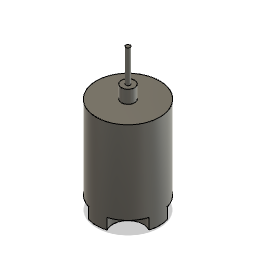
Motor v1 (Autodesk Fusion 360 design; units mm, degrees)
Autodesk Fusion 360 part; units mm, degrees
note: some values were not read from the file. Set by a fixed rule: which sketch regions a step uses.
sketch "Sketch1" plane through (0, 0, 0) normal (0, 1, 0) x (1, 0, 0)
  circle A0 centre (0, 0) radius 14.5
  dimension "d1" = 29
  constraint coincident A0.centre origin
  measures "d1" diameter of A0
extrude "Extrude1" add sketch "Sketch1" along normal blind 5
sketch "Sketch2" plane through (0, 0, 0) normal (0, -1, 0) x (1, 0, 0)
  circle A0 centre (0, 0) radius 14.5
  circle A1 centre (0, 0) radius 1.5
  circle A2 centre (0, 0) radius 14.5
  dimension "d4" = 3
  constraint coincident A0.centre A1.centre
  measures "d4" diameter of A1
extrude "Extrude2" add sketch "Sketch2" along normal blind 5 contours A0 A2 | A1
sketch "Sketch3" plane through (0, -5, 0) normal (0, -1, 0) x (1, 0, 0)
  circle A0 centre (0, 0) radius 14.5
  line L0 (0, 0) -> (10.253, 10.253)
  line L1 (0, 0) -> (14.5, 0) construction
  line L2 (0, 0) -> (10.253, -10.253)
  line L3 (0, 0) -> (-10.253, -10.253)
  line L4 (0, 0) -> (-10.253, 10.253)
  circle A1 centre (-10.253, -10.253) radius 7
  circle A2 centre (10.253, -10.253) radius 7
  circle A3 centre (10.253, 10.253) radius 7
  circle A4 centre (-10.253, 10.253) radius 7
  dimension "d7" = 45
  dimension "d8" = 14
  dimension "d9" = 14
  dimension "d10" = 14
  dimension "d11" = 14
  constraint horizontal L1
  constraint coincident A0.centre L0.start
  constraint coincident A0 L2.end
  constraint perpendicular L0 L2
  constraint coincident A0 L3.end
  constraint perpendicular L2 L3
  constraint coincident A0 L4.end
  constraint perpendicular L3 L4
  constraint coincident L3.end A1.centre
  constraint coincident L2.end A2.centre
  constraint coincident L0.end A3.centre
  constraint coincident L4.end A4.centre
  measures "d7" angle of L0 L1
  measures "d8" diameter of A1
  measures "d9" diameter of A2
  measures "d10" diameter of A3
  measures "d11" diameter of A4
extrude "Extrude3" cut sketch "Sketch3" against normal blind 5 contours A0 L0 A3 | A0 L2 A2 | A0 L0 A3 | A0 L2 A2 | A0 L4 A4 | A0 L3 A1 | A0 L3 A1 | A0 L4 A4
sketch "Sketch4" plane through (0, -5, 0) normal (0, -1, 0) x (1, 0, 0)
  arc A0 (-4.2549, -13.8617) -> (-13.8617, -4.2549) centre (-10.253, -10.253) ccw
  arc A1 (-4.2549, -13.8617) -> (4.2549, -13.8617) centre (0, 0) ccw
  arc A2 (13.8617, -4.2549) -> (4.2549, -13.8617) centre (10.253, -10.253) ccw
  arc A3 (13.8617, -4.2549) -> (13.8617, 4.2549) centre (0, 0) ccw
  arc A4 (4.2549, 13.8617) -> (13.8617, 4.2549) centre (10.253, 10.253) ccw
  arc A5 (4.2549, 13.8617) -> (-4.2549, 13.8617) centre (0, 0) ccw
  arc A6 (-13.8617, 4.2549) -> (-4.2549, 13.8617) centre (-10.253, 10.253) ccw
  arc A7 (-13.8617, 4.2549) -> (-13.8617, -4.2549) centre (0, 0) ccw
  circle A8 centre (0, 0) radius 1.5
  dimension "d14" = 3
  constraint coincident A1.centre A3.centre
  measures "d14" diameter of A8
extrude "Extrude4" add sketch "Sketch4" along normal blind 1 contours A8
sketch "Sketch5" plane through (0, 5, 0) normal (0, 1, 0) x (-1, 0, 0)
  circle A0 centre (0, 0) radius 14.5
  circle A1 centre (0, 0) radius 14.5
  constraint coincident A0.centre A1.centre
extrude "Extrude5" add sketch "Sketch5" along normal blind 28
sketch "Sketch6" plane through (0, 33, 0) normal (0, 1, 0) x (-1, 0, 0)
  circle A0 centre (0, 0) radius 14.5
  circle A1 centre (0, 0) radius 14.5
  constraint coincident A0.centre A1.centre
extrude "Extrude6" add sketch "Sketch6" along normal blind 5
sketch "Sketch7" plane through (0, 38, 0) normal (0, 1, 0) x (-1, 0, 0)
  circle A0 centre (0, 0) radius 14.5
  line L0 (0, 0) -> (10.253, -10.253)
  line L1 (0, 0) -> (14.5, 0) construction
  line L2 (0, 0) -> (-10.253, -10.253)
  line L3 (0, 0) -> (14.5, 0) construction
  line L4 (0, 0) -> (-10.253, 10.253)
  line L5 (-10.253, 10.253) -> (-6.7175, 6.7175)
  line L6 (-10.253, -10.253) -> (-6.7175, -6.7175)
  line L7 (10.253, -10.253) -> (6.7175, -6.7175)
  line L8 (10.253, 10.253) -> (8.8388, 8.8388)
  circle A1 centre (0, 0) radius 3.5
  circle A2 centre (0, 0) radius 12.5
  circle A3 centre (0, 0) radius 3
  dimension "d21" = 45
  dimension "d22" = 14.5
  dimension "d23" = 135
  dimension "d25" = 5
  dimension "d26" = 5
  dimension "d27" = 5
  dimension "d28" = 2
  dimension "d29" = 7
  dimension "d30" = 6
  constraint horizontal L1
  constraint coincident A0.centre L0.start
  constraint horizontal L3
  constraint coincident A0 L4.end
  constraint perpendicular L2 L4
  constraint coincident A0 L8.start
  constraint parallel L4 L5
  constraint parallel L2 L6
  constraint parallel L0 L7
  constraint coincident L8.end A2
  constraint concentric A1 A3
  measures "d21" angle of L0 L1
  measures "d22" distance of A0.centre L0.end
  measures "d23" angle of L2 L3
  measures "d25" distance of L4.end L5.end
  measures "d26" distance of L2.end L6.end
  measures "d27" distance of L0.end L7.end
  measures "d28" distance of L8.start L8.end
  measures "d29" diameter of A1
  measures "d30" diameter of A3
extrude "Extrude7" add sketch "Sketch7" along normal blind 6 contours L0 L2 A3 | L0 L4 A3 | L2 L4 A3
sketch "Sketch8" plane through (0, 44, 0) normal (0, 1, 0) x (-1, 0, 0)
  circle A0 centre (0, 0) radius 3
  circle A1 centre (0, 0) radius 1
  dimension "d33" = 2
  constraint coincident A0.centre A1.centre
  measures "d33" diameter of A1
extrude "Extrude8" add sketch "Sketch8" along normal blind 15 contours A1
equation "d8 = 0.7 cm * 2"
equation "d23 = 90 deg + 45 deg"
